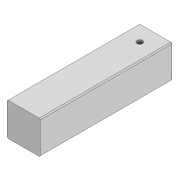
# Autodesk Inventor part: Stütze mitte
Saved by Autodesk Inventor 2020 (Build 240168000, 168)
## iProperties
Created: 2021-06-23
Part Number: Stütze mitte
Material: Generisch
Document SubType Name: Modeling
Designer: mike8
Density: 1 g/cm^3
Appearance: Vorgabe
Author: mike8
Autodesk Inventor part; units mm, degrees
ref_plane "YZ Plane" through (0, 0, 0) normal (1, 0, 0) x (0, 1, 0)
ref_plane "XZ Plane" through (0, 0, 0) normal (0, 1, 0) x (-1, 0, 0)
ref_plane "XY Plane" through (0, 0, 0) normal (0, 0, 1) x (1, 0, 0)
sketch "Skizze1" plane through (0, 0, 0) normal (0, 0, 1) x (1, 0, 0)
  line L0 (-18.741, 0) -> (23.259, 0) projected
  line L1 (0, -22.9262) -> (0, 19.0738) projected
  line L2 (-12.741, 13.0738) -> (17.259, 13.0738)
  line L3 (17.259, 13.0738) -> (17.259, -16.9262)
  line L4 (17.259, -16.9262) -> (-12.741, -16.9262)
  line L5 (-12.741, -16.9262) -> (-12.741, 13.0738)
  point P0 (0, 0)
  dimension "d0" = 30
  dimension "d1" = 30
  constraints: 8 end point, 2 parallel, 1 horizontal, 1 perpendicular
  measures "d0" distance of L2.start L2.end
  measures "d1" distance of L2.end L3.end
extrude "Extrusion1" add sketch "Skizze1" along normal blind 120
sketch "Skizze2" plane through (-12.741, 13.0738, 0) normal (0, 1, 0) x (1, 0, 0)
  line L0 (0, 0) -> (0, -120) projected
  line L1 (30, 0) -> (0, 0) projected
  point P0 (12.741, 0)
  point P1 (15, -15)
  dimension "d4" = 15
  dimension "d5" = 15
  measures "d4" distance from line of L0 point (15, -15)
  measures "d5" distance from line of point (15, -15) L1
hole "Bohrung1" at (2.259, 13.0738, 15) direction (0, -1, 0) diameter 5 end through all
chamfer "Fase1" distance 1 angle 45 8 edges at (17.259, 13.0738, 60) (-12.741, 13.0738, 60) (2.259, 13.0738, 0) (17.259, -1.9262, 0) (2.259, -16.9262, 0) (-12.741, -1.9262, 0) (17.259, -16.9262, 60) (-12.741, -16.9262, 60)
